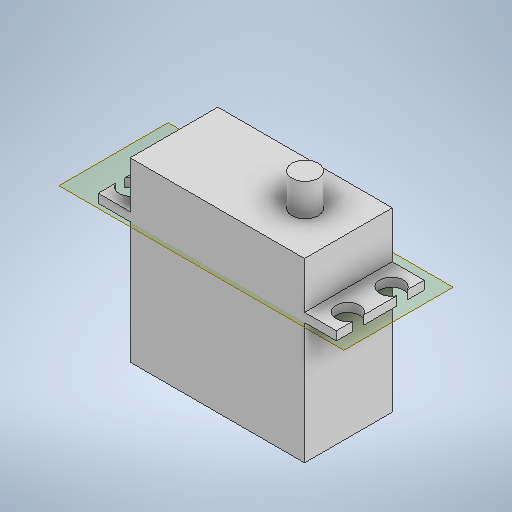
# Autodesk Inventor part: sarvo_motor
Saved by Autodesk Inventor 2025.1 (Build 291241000, 241)
## iProperties
Created: 2024-11-11
Part Number: sarvo_motor
Material: 一般
Document SubType Name: Modeling
Designer: dell
Density: 1 g/cm^3
Appearance: 既定
Author: dell
Autodesk Inventor part; units mm, degrees
ref_plane "YZ Plane" through (0, 0, 0) normal (1, 0, 0) x (0, 1, 0)
ref_plane "XZ Plane" through (0, 0, 0) normal (0, 1, 0) x (-1, 0, 0)
ref_plane "XY Plane" through (0, 0, 0) normal (0, 0, 1) x (1, 0, 0)
sketch "スケッチ1" plane through (0, 0, 0) normal (0, 1, 0) x (-1, 0, 0)
  line L0 (0, 0) -> (39.83, 0)
  line L1 (39.83, 0) -> (39.83, -20.04)
  line L2 (39.83, -20.04) -> (0, -20.04)
  line L3 (0, -20.04) -> (0, 0)
  dimension "d0" = 39.83
  dimension "d1" = 20.04
  constraints: 8 end point, 2 parallel, 1 horizontal, 1 perpendicular
  measures "d0" distance of L1.end L2.end
  measures "d1" distance of L2.end L0.start
extrude "押し出し1" add sketch "スケッチ1" along normal blind 40.4
ref_plane "作業平面2" through (0, 27.76, 0) normal (0, -1, 0) x (1, 0, 0)
sketch "スケッチ3" plane through (0, 27.76, 0) normal (0, -1, 0) x (1, 0, 0)
  line L0 (0, 0) -> (7.275, 0)
  line L1 (7.275, 0) -> (7.275, -20.0108)
  line L2 (7.275, -20.0108) -> (0, -20.0108)
  line L3 (0, -20.0108) -> (0, 0)
  line L4 (-39.83, -20.04) -> (-39.83, 0) projected
  line L5 (-39.83, 0) -> (-47.105, 0)
  line L6 (-47.105, 0) -> (-47.105, -20.04)
  line L7 (-47.105, -20.04) -> (-39.83, -20.04)
  line L8 (-39.83, -20.04) -> (-39.83, 0)
  dimension "d5" = 7.275
  dimension "d6" = 20.0108
  dimension "d7" = 7.275
  constraints: 16 end point, 4 parallel, 2 horizontal, 2 perpendicular
  measures "d5" distance of L1.end L2.end
  measures "d6" distance of L0.end L1.end
  measures "d7" distance of L7.end L6.end
extrude "押し出し2" add sketch "スケッチ3" against normal blind 2
sketch "スケッチ6" plane through (0, 40.4, 0) normal (0, 1, 0) x (1, 0, 0)
  line L0 (0, 0) -> (0, 20.04) projected
  line L1 (0, 0) -> (0, 20.04) projected
  line L2 (-39.83, 20.04) -> (-39.83, 0) projected
  line L3 (-39.83, 10.02) -> (0, 10.02)
  circle A0 centre (-9.9, 10.02) radius 3
  dimension "d11" = 9.9
  dimension "d12" = 6
  constraints: 4 midpoint, 2 end point, 1 centre point, 1 coincident, 1 horizontal, 1 perpendicular
  measures "d11" distance of point (0, 10.02) point (-9.9, 10.02)
  measures "d12" diameter of A0
extrude "押し出し3" add sketch "スケッチ6" along normal blind 7.4
sketch "スケッチ9" plane through (0, 29.76, 0) normal (0, 1, 0) x (1, 0, 0)
  circle A0 centre (-44.6339, 15.02) radius 2.75
  circle A1 centre (-44.6339, 5.02) radius 2.75
  circle A2 centre (4.8661, 15.0054) radius 2.75
  circle A3 centre (4.8661, 5.0054) radius 2.75
  line L0 (-47.105, 0) -> (-47.105, 20.04) projected
  line L1 (-47.105, 10.02) -> (-39.83, 10.02)
  line L2 (-39.83, 20.04) -> (-39.83, 0) projected
  line L3 (-47.105, 20.04) -> (-47.105, 0) projected
  line L4 (-44.6339, 15.02) -> (-44.6339, 5.02)
  line L5 (4.8661, 15.0054) -> (4.8661, 5.0054)
  line L6 (7.275, 20.0108) -> (7.275, 0) projected
  line L7 (7.275, 10.0054) -> (0.184, 10.0054)
  point P0 (0, 0)
  point P1 (-44.6339, 10.02)
  point P2 (4.8661, 10.0054)
  dimension "d15" = 10
  dimension "d16" = 5.5
  dimension "d17" = 5.5
  dimension "d18" = 5.5
  dimension "d19" = 10
  dimension "d20" = 5.5
  dimension "d21" = 49.5
  constraints: 8 end point, 5 midpoint, 4 centre point, 2 perpendicular, 2 point on line, 1 horizontal, 1 vertical
  measures "d15" distance of L4.end L4.start
  measures "d16" diameter of A1
  measures "d17" diameter of A2
  measures "d18" diameter of A3
  measures "d19" distance of L5.end L5.start
  measures "d20" diameter of A0
  measures "d21" distance of L5.start L4.start
hole "穴1" at (-44.6339, 29.76, -15.02) at (4.8661, 29.76, -15.0054) at (-44.6339, 29.76, -5.02) at (4.8661, 29.76, -5.0054) direction (0, -1, 0) diameter 5.4 end through all
